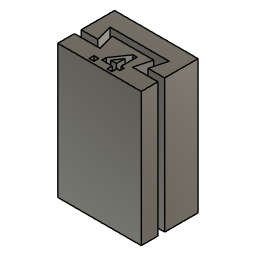
Test_Andorinha (Autodesk Fusion 360 design; units mm, degrees)
Autodesk Fusion 360 part; units mm, degrees
sketch "Esboço1" plane through (0, 0, 0) normal (0, 0, 1) x (1, 0, 0)
  line L0 (5, 0) -> (5, -1)
  line L1 (0, -1) -> (0, 0)
  line L2 (5, 0) -> (5, 1)
  line L3 (5, 1) -> (0, 1)
  line L4 (0, 1) -> (0, 0)
  line L5 (4, -1) -> (4.2679, 0)
  line L6 (4, -1) -> (5, -1) construction
  line L7 (2.5, 1) -> (2.5, 0.0017)
  line L8 (1, -1) -> (0.7321, 0)
  line L9 (4, -1) -> (5, -1)
  line L10 (1, -1) -> (0.7321, 0)
  line L11 (1, -1) -> (0, -1)
  line L12 (0.7321, 0) -> (4.2679, 0)
  line L13 (1.5213, -1.4) -> (0, -1.4)
  line L14 (1.5213, -1.4) -> (1.2533, -0.4)
  line L15 (1.2533, -0.4) -> (3.7467, -0.4)
  line L16 (3.4787, -1.4) -> (3.7467, -0.4)
  line L17 (3.4787, -1.4) -> (5, -1.4)
  line L18 (0, -1.4) -> (0, -2.4)
  line L19 (0, -2.4) -> (5, -2.4)
  line L20 (5, -2.4) -> (5, -1.4)
  line L21 (1.2327, -2.627) -> (3.7601, -2.635) construction
  line L22 (3.7601, -2.635) -> (3.7673, -0.373) construction
  line L23 (3.7673, -0.373) -> (1.2399, -0.365) construction
  line L24 (1.2399, -0.365) -> (1.2327, -2.627) construction
  dimension "d1" = 5
  dimension "d2" = 1
  dimension "d3" = 1
  dimension "d4" = 75
  dimension "d5" = 1
  dimension "d6" = -0.4
  dimension "d7" = 1
  dimension "d8" = 1.5
  dimension "d14" = 1
  dimension "d15" = 1
  dimension "d16" = 1
  text T0 ".4" font "Arial" height 1.5 bold align centre middle in box 2.5274 x 2.262 at (1.2327, -2.627) x (0.999995, -0.003158) y (0.003158, 0.999995) spacing 1
  constraint vertical L0
  constraint vertical L1
  constraint coincident L1.end L4.end
  constraint vertical L2
  constraint horizontal L3
  constraint vertical L4
  constraint horizontal L6
  constraint midpoint L3 L7.start
  constraint symmetric L5.start L7 L8.start
  constraint symmetric L5.end L7 L8.end
  constraint symmetric L0.end L7 L1.start
  constraint horizontal L12
  constraint perpendicular L13 L18
  constraint perpendicular L18 L19
  constraint equal L3 L19
  constraint coincident L0.start L2.start
  measures "d1" distance of L1.end L0.start
  measures "d2" distance of L1.end L1.start
  measures "d3" distance of L1.end L3.end
  measures "d4" angle of L5 L6
  measures "d5" distance of L0.end L5.start
  measures "d7" distance of L13.end L18.end
  measures "d14" distance of L0.start L2.end
  measures "d15" distance of L0.start L0.end
  measures "d16" distance of L3 L5.end
extrude "Extrusão1" add sketch "Esboço1" along normal blind 8 makes body 1 at (1.6667, -2.4, 2.6667) makes body 2 at (4.1667, 1, 2.6667)
extrude "Extrusão2" cut sketch "Esboço1" against normal blind 1 from surface at 8 text T0 bodies 1
equation "d2 = d1 * 0.2"
equation "d3 = d14"
equation "d5 = d1 * 0.2"
equation "d7 = d1 * 0.2"
equation "d14 = d1 * 0.2"
equation "d15 = d2"
equation "d16 = d14"
named bodies: "Macho", "Femea"
